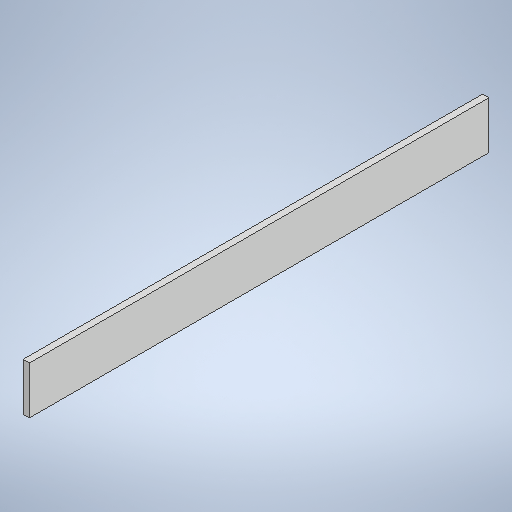
# Autodesk Inventor part: TapaLateral
Saved by Autodesk Inventor 2025 (Build 290162000, 162)
## iProperties
Created: 2024-11-21
Part Number: TapaLateral
Material: Generic
Document SubType Name: Sheet Metal
Designer: g.marin
Density: 1 g/cm^3
Sheet Metal Rule: Default
Appearance: Default
Author: g.marin
Autodesk Inventor part; units mm, degrees
ref_plane "YZ Plane" through (0, 0, 0) normal (1, 0, 0) x (0, 1, 0)
ref_plane "XZ Plane" through (0, 0, 0) normal (0, 1, 0) x (-1, 0, 0)
ref_plane "XY Plane" through (0, 0, 0) normal (0, 0, 1) x (1, 0, 0)
sketch "Sketch1" plane through (0, 0, 0) normal (1, 0, 0) x (0, 1, 0)
  line L0 (-11.25, 108.75) -> (11.25, 108.75)
  line L1 (11.25, 108.75) -> (11.25, -108.75)
  line L2 (11.25, -108.75) -> (-11.25, -108.75)
  line L3 (-11.25, -108.75) -> (-11.25, 108.75)
  line L4 (-11.25, 108.75) -> (11.25, -108.75) construction
  line L5 (11.25, 108.75) -> (-11.25, -108.75) construction
  point P0 (0, 0)
  dimension "d0" = 217.5
  dimension "d1" = 22.5
  constraints: 12 end point, 2 midpoint, 2 parallel, 1 horizontal, 1 perpendicular
  measures "d0" distance of L0.end L1.end
  measures "d1" distance of L1.end L2.end
extrude "Extrusion1" add sketch "Sketch1" along normal blind 3
equation "\"BendRadius\" = Thickness"
equation "\"BendReliefWidth\" = Thickness"
equation "\"BendReliefDepth\" = 0.5 * Thickness"
equation "\"CornerReliefSize\" = 4 * Thickness"
equation "\"MinimumRemnant\" = 2 * Thickness"
equation "\"TransitionRadius\" = BendRadius"
equation "\"JacobiRadiusSize\" = BendRadius"
equation "\"GapSize\" = Thickness"
equation "\"Thickness\" = 3.048"
body "Solid1"
